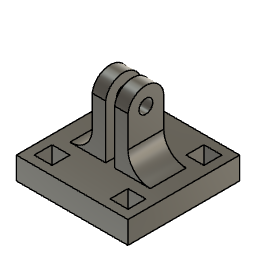
BigCameraMountBase v7 (Autodesk Fusion 360 design; units mm, degrees)
Autodesk Fusion 360 part; units mm, degrees
sketch "Sketch1" plane through (0, 0, 0) normal (0, 1, 0) x (1, 0, 0)
  line L0 (0, 0) -> (25, 0)
  line L1 (25, 0) -> (25, -5)
  line L2 (25, -5) -> (0, -5)
  line L3 (0, -5) -> (0, 0)
  dimension "d1" = 25
  dimension "d2" = 5
  constraint horizontal L0
  constraint vertical L1
  constraint horizontal L2
  constraint vertical L3
  constraint coincident L0.start L3.end
  measures "d1" distance of L0.start L0.end
  measures "d2" distance of L0.start L2.end
extrude "Extrude1" add sketch "Sketch1" along normal blind 25
hole "Hole2" at (19.9955, 4.9703, 5) direction (0, 0, -1) diameter 6 depth 9 tip angle 118
hole "Hole3" at (19.9612, 19.927, 5) direction (0, 0, -1) diameter 6 depth 9 tip angle 118
hole "Hole4" at (5.0045, 19.9955, 5) direction (0, 0, -1) diameter 6 depth 9 tip angle 118
hole "Hole5" at (5.0388, 4.9361, 5) direction (0, 0, -1) diameter 6 depth 9 tip angle 118
sketch "Sketch8" plane through (0, 0, 5) normal (0, 0, 1) x (-1, 0, 0)
  circle A0 centre (-5.0388, -4.9361) radius 3
  circle A1 centre (-5.0045, -19.9955) radius 3
  circle A2 centre (-19.9612, -19.927) radius 3
  circle A3 centre (-19.9955, -4.9703) radius 3
  line L0 (0, 0) -> (-25, 0)
  line L1 (-25, 0) -> (-25, -25)
  line L2 (-25, -25) -> (0, -25)
  line L3 (0, -25) -> (0, 0)
  line L4 (-8.5, -16.5) -> (-16.5, -16.5)
  line L5 (-16.5, -16.5) -> (-16.5, -8.5)
  line L6 (-16.5, -8.5) -> (-8.5, -8.5)
  line L7 (-8.5, -8.5) -> (-8.5, -16.5)
  line L8 (-8.5, -16.5) -> (-11.5, -16.5)
  line L9 (-11.5, -16.5) -> (-11.5, -8.5)
  line L10 (-11.5, -8.5) -> (-8.5, -8.5)
  line L11 (-8.5, -8.5) -> (-8.5, -16.5)
  line L12 (-16.5, -16.5) -> (-13.5, -16.5)
  line L13 (-13.5, -16.5) -> (-13.5, -8.5)
  line L14 (-13.5, -8.5) -> (-16.5, -8.5)
  line L15 (-16.5, -8.5) -> (-16.5, -16.5)
  constraint horizontal L4
  constraint vertical L5
  constraint horizontal L6
  constraint vertical L7
  constraint horizontal L8
  constraint vertical L9
  constraint horizontal L10
  constraint vertical L11
  constraint horizontal L12
  constraint vertical L13
  constraint horizontal L14
  constraint vertical L15
  constraint coincident L6 L13.end
extrude "Extrude5" add sketch "Sketch8" along normal blind 12 contours L4 L6 L7 L8 L9 L10 L11 | L4 L5 L6 L12 L13 L14 L15
sketch "Sketch9" plane through (16.5, 0, 0) normal (1, 0, 0) x (0, 1, 0)
  line L0 (8.5, 5) -> (16.5, 5)
  line L1 (16.5, 5) -> (16.5, 17)
  line L2 (16.5, 17) -> (8.5, 17)
  line L3 (8.5, 17) -> (8.5, 5)
  arc A0 (16.5, 17) -> (8.5, 17) centre (12.5, 16.4643) ccw
  constraint coincident L1.end L2.start
  constraint coincident L2.end L3.start
extrude "Extrude6" add sketch "Sketch9" against normal blind 3 contours L2 A0
sketch "Sketch10" plane through (8.5, 0, 0) normal (-1, 0, 0) x (0, -1, 0)
  line L0 (-16.5, 5) -> (-8.5, 5)
  line L1 (-8.5, 5) -> (-8.5, 17)
  line L2 (-8.5, 17) -> (-16.5, 17)
  line L3 (-16.5, 17) -> (-16.5, 5)
  arc A0 (-8.5, 17) -> (-16.5, 17) centre (-12.5, 16.4643) ccw
  constraint coincident L1.end L2.start
  constraint coincident L2.end L3.start
extrude "Extrude7" add sketch "Sketch10" against normal blind 3 contours L2 A0
fillet "Fillet1" radius 5 1 edges at (16.5, 12.5, 5)
fillet "Fillet2" radius 5 1 edges at (8.5, 12.5, 5)
hole "Hole7" at (16.5, 12.5, 16.4643) direction (-1, 0, 0) diameter 3.1 depth 10 tip angle 118
delete_face "DeleteFace1" 1 faces at (20.145, 1.974, 3.3333)
delete_face "DeleteFace2" 1 faces at (20.1108, 16.9308, 3.3333)
delete_face "DeleteFace3" 1 faces at (5.1883, 1.9398, 3.3333)
delete_face "DeleteFace4" 1 faces at (5.1541, 16.9992, 3.3333)
sketch "Sketch11" plane through (0, 0, 5) normal (0, 0, 1) x (-1, 0, 0)
  line L0 (-3.5, -16.5) -> (-11.5, -16.5)
  line L1 (-11.5, -16.5) -> (-11.5, -8.5)
  line L2 (-11.5, -8.5) -> (-3.5, -8.5)
  line L3 (-3.5, -8.5) -> (-3.5, -16.5)
  line L4 (-21.5, -8.5) -> (-13.5, -8.5)
  line L5 (-13.5, -8.5) -> (-13.5, -16.5)
  line L6 (-13.5, -16.5) -> (-21.5, -16.5)
  line L7 (-21.5, -16.5) -> (-21.5, -8.5)
  line L8 (0, 0) -> (-25, 0)
  line L9 (-25, 0) -> (-25, -25)
  line L10 (-25, -25) -> (0, -25)
  line L11 (0, -25) -> (0, 0)
  line L12 (-2, -2) -> (-6, -2)
  line L13 (-6, -2) -> (-6, -6)
  line L14 (-6, -6) -> (-2, -6)
  line L15 (-2, -6) -> (-2, -2)
  line L16 (-6, -2) -> (-6, -6)
  line L17 (-23, -2) -> (-19, -2)
  line L18 (-19, -2) -> (-19, -6)
  line L19 (-19, -6) -> (-23, -6)
  line L20 (-23, -6) -> (-23, -2)
  line L21 (-23, -23) -> (-19, -23)
  line L22 (-19, -23) -> (-19, -19)
  line L23 (-19, -19) -> (-23, -19)
  line L24 (-23, -19) -> (-23, -23)
  line L25 (-2, -23) -> (-6, -23)
  line L26 (-6, -23) -> (-6, -19)
  line L27 (-6, -19) -> (-2, -19)
  line L28 (-2, -19) -> (-2, -23)
  constraint horizontal L12
  constraint vertical L13
  constraint horizontal L14
  constraint vertical L15
  constraint vertical L16
  constraint horizontal L17
  constraint vertical L18
  constraint horizontal L19
  constraint vertical L20
  constraint horizontal L21
  constraint vertical L22
  constraint horizontal L23
  constraint vertical L24
  constraint horizontal L25
  constraint vertical L26
  constraint horizontal L27
  constraint vertical L28
extrude "Extrude8" cut sketch "Sketch11" against normal blind 5 contours L12 L13 L14 L15 L16 | L17 L18 L19 L20 | L21 L22 L23 L24 | L25 L26 L27 L28
